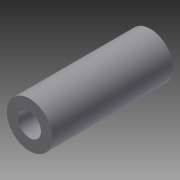
# Autodesk Inventor part: POST0.5625-0.625-bif
Saved by Autodesk Inventor 2014 SP2 (Build 180246200, 246)
## iProperties
Created: 2020-02-04
Part Number: POST0.5625-0.625-bif
Material: Generic
Catalog Web Link: www.cadenas.de
Description: BIF Post-Bimba FLAT-1
Vendor: BIMBA
Document SubType Name: Modeling
Designer: psadmin
Manufacturer: BIMBA
Mass: 0.332224 g
Surface Area: 4.89024 cm^2
Volume: 0.332224 cm^3
Density: 1 g/cm^3
Appearance: PSOLRGB-192-192-192
Category: PARTsolutions
Company: BIMBA
Title: POST0.5625-0.625-bif
Author: Cadenas PARTsolutions
Comments: Bimba FLAT-1
PSOL_IDENT_0: {$CADENAS_DATA\23d-libs\bimba\bimba_brand\bimba_imperial\bimba_full_line\flat_cylinders\fo1\bif_post
PSOL_IDENT_1: .prj},187 {VTYP=3D},{NB=POST0.5625-0.625-bif},{LINA=POST0.5625-0.625-bif},{NN=BIF Post},{DATE=22.01.
PSOL_IDENT_2: 2020 09:06:04},{GEOMDATE=09.03.2017 10:15:08},{VERSION=},{LINEID=10},{WBVAR=L,AB},{WBNUMERIC=L}  {NB=
PSOL_IDENT_3: POST0.5625-0.625-bif},{LINA=POST0.5625-0.625-bif},{KT=DUMMY},{PN=POST0.5625-0.625},{BORE=0.5625},{L=
PSOL_IDENT_4: 0.62500},{AB=},{DIA=0.235},{ID=0.11800}
NN: BIF Post
NT: Bimba FLAT-1
NB: POST0.5625-0.625-bif
NBSYN: $PN.-bif
LINA: POST0.5625-0.625-bif
PN: POST0.5625-0.625
BORE: 0.5625
L: 0.625
AB: Standard
SUPPLIER: BIMBA
ARTICLENO: POST0.5625-0.625-bif
BOMINFO: POST0.5625-0.625-bif
CREATOR: CADENAS GmbH
Autodesk Inventor part; units mm, degrees
sketch "Sketch_1" plane through (0, 0, 0) normal (1, 0, 0) x (0, 1, 0)
  line L0 (0, -15.875) -> (0, 0)
  line L1 (0, 0) -> (2.9845, 0)
  line L2 (2.9845, 0) -> (2.9845, -15.875)
  line L3 (2.9845, -15.875) -> (0, -15.875)
  line L4 (0, -15.875) -> (0, 0)
  constraints: 10 end point
revolve "Revolution1" add sketch "Sketch_1" angle 360 about axis through (0, 0, -15.875) along (0, 0, -1)
sketch "Sketch2" plane through (0, 0, 0) normal (0, 0, 1) x (1, 0, 0)
  point P0 (0, 0)
hole "Hole1" at (0, 0, 0) direction (0, 0, -1) diameter 2.9972 depth 15.875
ref_plane "screw_XY" through (0, 0, 0) normal (0, 0, 1) x (1, 0, 0)
ref_plane "screw_YZ" through (0, 0, 0) normal (1, 0, 0) x (0, 1, 0)
ref_plane "screw_ZX" through (0, 0, 0) normal (0, 1, 0) x (0, 0, 1)
body "Solid1"
